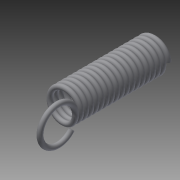
# Autodesk Inventor part: Spring2
Saved by Autodesk Inventor 2013 (Build 170138000, 138)
## iProperties
Created: 2012-10-29
Part Number: Spring2
Material: Generic
Document SubType Name: Modeling
Designer: uqgtayle
Density: 1 g/cm^3
Author: uqgtayle
Autodesk Inventor part; units mm, degrees
ref_plane "XZ Plane" through (0, 0, 0) normal (0, 1, 0) x (-1, 0, 0)
ref_plane "XY Plane" through (0, 0, 0) normal (0, 0, 1) x (1, 0, 0)
sketch "Sketch1" plane through (0, 0, 0) normal (0, 0, 1) x (1, 0, 0)
  circle A0 centre (1.9, 0) radius 0.335
  point P0 (0, 0)
  dimension "d2" = 0.67
  dimension "d4" = 1.9
  constraints: 1 centre point
  measures "d2" diameter of A0
  measures "d4" distance of point (0, 0) A0.centre
coil "Coil1" sketch "Sketch1" operation add axis through (0, -10, 0) along (0, 1, 0) pitch 0.7 turns 18 hand right
ref_plane "Work Plane2" through (2.1, 0, 0) normal (1, 0, 0) x (0, 1, 0)
sketch "Sketch6" plane through (1.9, 0, 0) normal (0, 0, 1) x (1, 0, 0)
  circle A0 centre (0, 0) radius 0.335 projected
  point P0 (0.335, 0)
  point P1 (-1.9, 0)
  constraints: 1 horizontal alignment
sketch "Sketch8" plane through (2.1, 0, 0) normal (1, 0, 0) x (0, 1, 0)
  arc A0 (-0.0034, 0) -> (-0.5207, -1.4884) centre (-2.4034, 0) ccw
  line L0 (-2.4034, 0) -> (0.613, 0) construction
  line L1 (0.613, 0) -> (-2.4034, 0) construction
  line L2 (-2.4034, 0) -> (0.1548, -2.0224) construction
  point P0 (0, 0)
  dimension "d16" = 4.8
  constraints: 6 end point, 2 point on circle, 2 point on line, 1 centre point, 1 collinear, 1 horizontal
  measures "d16" diameter of A0
sweep "Sweep1" add profiles "Sketch6" path "Sketch8"
body "Solid1"
